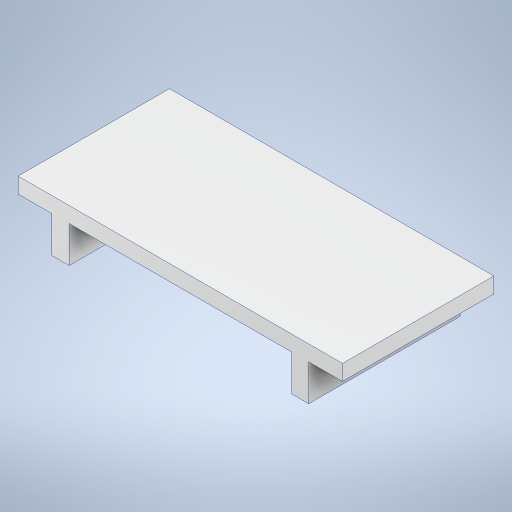
# Autodesk Inventor part: ZadBabkaOsnova
Saved by Autodesk Inventor 2024 (Build 280153000, 153)
## iProperties
Created: 2023-08-28
Part Number: ZadBabkaOsnova
Material: Aluminum 6061
Document SubType Name: Modeling
Designer: KirikDK
Density: 2.7 g/cm^3
Appearance: Aluminum - Flat
Mass: 3033.45 g
Surface Area: 1818.9 cm^2
Volume: 1123.5 cm^3
Author: KirikDK
Autodesk Inventor part; units mm, degrees
ref_plane "YZ Plane" through (0, 0, 0) normal (1, 0, 0) x (0, 1, 0)
ref_plane "XZ Plane" through (0, 0, 0) normal (0, 1, 0) x (-1, 0, 0)
ref_plane "XY Plane" through (0, 0, 0) normal (0, 0, 1) x (1, 0, 0)
sketch "Sketch1" plane through (0, 0, 0) normal (0, 1, 0) x (-1, 0, 0)
  line L0 (50, 50) -> (-125, 50)
  line L1 (-125, 50) -> (-125, -125)
  line L2 (-125, -125) -> (50, -125)
  line L3 (50, -125) -> (50, 50)
  point P0 (0, 0)
  dimension "d0" = 175
  dimension "d1" = 175
  constraints: 8 end point, 2 parallel, 1 horizontal, 1 perpendicular
  measures "d0" distance of L2.end L0.start
  measures "d1" distance of L0.start L0.end
extrude "Extrusion1" add sketch "Sketch1" along normal blind 12
sketch "Sketch2" plane through (0, 12, 0) normal (0, 1, 0) x (1, 0, 0)
  line L0 (-50, -50) -> (125, -50) projected
  line L1 (-150, -50) -> (225, -50)
  line L2 (225, -50) -> (225, 125)
  line L3 (225, 125) -> (-150, 125)
  line L4 (-150, 125) -> (-150, -50)
  line L5 (-50, 125) -> (-50, -50) projected
  line L6 (125, -50) -> (125, 125) projected
  point P0 (0, 0)
  point P1 (55, -50)
  dimension "d8" = 100
  dimension "d9" = 100
  constraints: 8 end point, 2 parallel, 1 horizontal, 1 perpendicular, 1 point on line
  measures "d8" distance between parallel lines of L6 L2
  measures "d9" distance between parallel lines of L5 L4
extrude "Extrusion2" add sketch "Sketch2" against normal blind 18
sketch "Sketch3" plane through (0, 0, 0) normal (0, -1, 0) x (1, 0, 0)
  line L0 (225, 50) -> (-150, 50) projected
  line L1 (-150, 50) -> (-150, -125) projected
  line L2 (-150, -125) -> (225, -125) projected
  line L3 (225, -125) -> (225, 50) projected
  line L4 (-110.9465, 50) -> (-90.9465, 50)
  line L5 (-90.9465, 50) -> (-90.9465, -125)
  line L6 (-90.9465, -125) -> (-110.9465, -125)
  line L7 (-110.9465, -125) -> (-110.9465, 50)
  line L8 (185.9465, 50) -> (165.9465, 50)
  line L9 (165.9465, 50) -> (165.9465, -125)
  line L10 (165.9465, -125) -> (185.9465, -125)
  line L11 (185.9465, -125) -> (185.9465, 50)
  point P0 (0, 0)
  dimension "d10" = 256.893
  dimension "d11" = 20
  dimension "d12" = 20
  dimension "d13" = 39.0535
  dimension "d14" = 39.0535
  constraints: 16 end point, 4 parallel, 4 point on line, 2 horizontal, 2 perpendicular
  measures "d10" distance between parallel lines of L9 L5
  measures "d11" distance between parallel lines of L5 L7
  measures "d12" distance between parallel lines of L11 L9
  measures "d13" distance between parallel lines of L3 L11
  measures "d14" distance between parallel lines of L1 L7
extrude "Extrusion3" add sketch "Sketch3" along normal blind 48 contours L11 L2 L9 L0 | L5 L2 L7 L0
body "Solid1"
